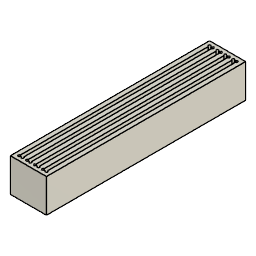
PCB Tolerance Tester (Autodesk Fusion 360 design; units mm, degrees)
Autodesk Fusion 360 part; units mm, degrees
sketch "Sketch1" plane through (0, 0, 0) normal (0, 0, 1) x (1, 0, 0)
  arc A0 (-0.5916, 85.05) -> (-0.493, 85.1333) centre (-0.5916, 85.15) ccw
  line L0 (-0.5916, 85.05) -> (-0.9084, 85.05)
  arc A1 (-1.007, 85.1333) -> (-1.5833, 84.557) centre (-1.5, 85.05) ccw
  arc A2 (0.0833, 84.557) -> (-0.493, 85.1333) centre (0, 85.05) ccw
  arc A3 (-1.007, 85.1333) -> (-0.9084, 85.05) centre (-0.9084, 85.15) ccw
  arc A4 (-1.5, 84.4584) -> (-1.5833, 84.557) centre (-1.6, 84.4584) ccw
  line L1 (-1.5, 84.4584) -> (-1.5, 0.5916)
  line L2 (0, 0.5916) -> (0, 84.4584)
  arc A5 (0.0833, 84.557) -> (0, 84.4584) centre (0.1, 84.4584) ccw
  line L3 (-1.5, 42.525) -> (0, 42.525) construction
  arc A6 (0, 0.5916) -> (0.0833, 0.493) centre (0.1, 0.5916) ccw
  arc A7 (-1.5833, 0.493) -> (-1.5, 0.5916) centre (-1.6, 0.5916) ccw
  arc A8 (-0.9084, 0) -> (-1.007, -0.0833) centre (-0.9084, -0.1) ccw
  arc A9 (-1.5833, 0.493) -> (-1.007, -0.0833) centre (-1.5, 0) ccw
  line L4 (-0.5916, 0) -> (-0.9084, 0)
  arc A10 (-0.493, -0.0833) -> (-0.5916, 0) centre (-0.5916, -0.1) ccw
  arc A11 (-0.493, -0.0833) -> (0.0833, 0.493) centre (0, 0) ccw
  line L5 (-3.5, 87.05) -> (12.65, 87.05)
  line L6 (12.65, 87.05) -> (12.65, -2)
  line L7 (12.65, -2) -> (-3.5, -2)
  line L8 (-3.5, -2) -> (-3.5, 87.05)
  line L9 (2.9334, 0) -> (2.5916, 0)
  line L10 (2, 84.4584) -> (2, 0.5916)
  arc A12 (3.6083, 84.557) -> (3.525, 84.4584) centre (3.625, 84.4584) ccw
  arc A13 (2.9334, 85.05) -> (3.032, 85.1333) centre (2.9334, 85.15) ccw
  arc A14 (1.9167, 0.493) -> (2.493, -0.0833) centre (2, 0) ccw
  arc A15 (2.493, 85.1333) -> (2.5916, 85.05) centre (2.5916, 85.15) ccw
  arc A16 (3.032, -0.0833) -> (3.6083, 0.493) centre (3.525, 0) ccw
  arc A17 (2, 84.4584) -> (1.9167, 84.557) centre (1.9, 84.4584) ccw
  arc A18 (3.525, 0.5916) -> (3.6083, 0.493) centre (3.625, 0.5916) ccw
  line L11 (2.9334, 85.05) -> (2.5916, 85.05)
  arc A19 (2.5916, 0) -> (2.493, -0.0833) centre (2.5916, -0.1) ccw
  line L12 (2, 42.525) -> (3.525, 42.525) construction
  arc A20 (2.493, 85.1333) -> (1.9167, 84.557) centre (2, 85.05) ccw
  arc A21 (3.6083, 84.557) -> (3.032, 85.1333) centre (3.525, 85.05) ccw
  arc A22 (3.032, -0.0833) -> (2.9334, 0) centre (2.9334, -0.1) ccw
  arc A23 (1.9167, 0.493) -> (2, 0.5916) centre (1.9, 0.5916) ccw
  line L13 (3.525, 0.5916) -> (3.525, 84.4584)
  arc A24 (5.4417, 0.493) -> (6.018, -0.0833) centre (5.525, 0) ccw
  line L14 (10.65, 0.5916) -> (10.65, 84.4584)
  line L15 (7.075, 0.5916) -> (7.075, 84.4584)
  line L16 (9.075, 42.525) -> (10.65, 42.525) construction
  arc A25 (9.568, 85.1333) -> (8.9917, 84.557) centre (9.075, 85.05) ccw
  line L17 (5.525, 84.4584) -> (5.525, 0.5916)
  arc A26 (6.582, -0.0833) -> (7.1583, 0.493) centre (7.075, 0) ccw
  arc A27 (10.157, -0.0833) -> (10.7333, 0.493) centre (10.65, 0) ccw
  arc A28 (6.018, 85.1333) -> (5.4417, 84.557) centre (5.525, 85.05) ccw
  line L18 (10.0584, 85.05) -> (9.6666, 85.05)
  arc A29 (8.9917, 0.493) -> (9.075, 0.5916) centre (8.975, 0.5916) ccw
  line L19 (6.4834, 0) -> (6.1166, 0)
  arc A30 (6.018, 85.1333) -> (6.1166, 85.05) centre (6.1166, 85.15) ccw
  arc A31 (9.568, 85.1333) -> (9.6666, 85.05) centre (9.6666, 85.15) ccw
  arc A32 (7.075, 0.5916) -> (7.1583, 0.493) centre (7.175, 0.5916) ccw
  line L20 (5.525, 42.525) -> (7.075, 42.525) construction
  arc A33 (6.1166, 0) -> (6.018, -0.0833) centre (6.1166, -0.1) ccw
  arc A34 (7.1583, 84.557) -> (7.075, 84.4584) centre (7.175, 84.4584) ccw
  line L21 (6.4834, 85.05) -> (6.1166, 85.05)
  arc A35 (9.075, 84.4584) -> (8.9917, 84.557) centre (8.975, 84.4584) ccw
  line L22 (9.075, 84.4584) -> (9.075, 0.5916)
  arc A36 (10.7333, 84.557) -> (10.65, 84.4584) centre (10.75, 84.4584) ccw
  arc A37 (6.582, -0.0833) -> (6.4834, 0) centre (6.4834, -0.1) ccw
  arc A38 (8.9917, 0.493) -> (9.568, -0.0833) centre (9.075, 0) ccw
  arc A39 (6.4834, 85.05) -> (6.582, 85.1333) centre (6.4834, 85.15) ccw
  arc A40 (7.1583, 84.557) -> (6.582, 85.1333) centre (7.075, 85.05) ccw
  arc A41 (9.6666, 0) -> (9.568, -0.0833) centre (9.6666, -0.1) ccw
  arc A42 (10.7333, 84.557) -> (10.157, 85.1333) centre (10.65, 85.05) ccw
  line L23 (10.0584, 0) -> (9.6666, 0)
  arc A43 (5.525, 84.4584) -> (5.4417, 84.557) centre (5.425, 84.4584) ccw
  arc A44 (10.65, 0.5916) -> (10.7333, 0.493) centre (10.75, 0.5916) ccw
  arc A45 (10.157, -0.0833) -> (10.0584, 0) centre (10.0584, -0.1) ccw
  arc A46 (5.4417, 0.493) -> (5.525, 0.5916) centre (5.425, 0.5916) ccw
  arc A47 (10.0584, 85.05) -> (10.157, 85.1333) centre (10.0584, 85.15) ccw
  arc A48 (9.568, 85.1333) -> (9.6666, 85.05) centre (9.6666, 85.15) ccw
  arc A49 (6.4834, 85.05) -> (6.582, 85.1333) centre (6.4834, 85.15) ccw
  arc A50 (10.0584, 85.05) -> (10.157, 85.1333) centre (10.0584, 85.15) ccw
  arc A51 (6.018, 85.1333) -> (5.4417, 84.557) centre (5.525, 85.05) ccw
  line L24 (10.0584, 85.05) -> (9.6666, 85.05)
  arc A52 (2.9334, 85.05) -> (3.032, 85.1333) centre (2.9334, 85.15) ccw
  arc A53 (10.7333, 84.557) -> (10.157, 85.1333) centre (10.65, 85.05) ccw
  arc A54 (6.018, 85.1333) -> (6.1166, 85.05) centre (6.1166, 85.15) ccw
  arc A55 (5.525, 84.4584) -> (5.4417, 84.557) centre (5.425, 84.4584) ccw
  arc A56 (2, 84.4584) -> (1.9167, 84.557) centre (1.9, 84.4584) ccw
  arc A57 (0.0833, 84.557) -> (0, 84.4584) centre (0.1, 84.4584) ccw
  arc A58 (10.7333, 84.557) -> (10.65, 84.4584) centre (10.75, 84.4584) ccw
  arc A59 (-1.007, 85.1333) -> (-1.5833, 84.557) centre (-1.5, 85.05) ccw
  line L25 (2.9334, 85.05) -> (2.5916, 85.05)
  arc A60 (3.6083, 84.557) -> (3.032, 85.1333) centre (3.525, 85.05) ccw
  arc A61 (-1.007, 85.1333) -> (-0.9084, 85.05) centre (-0.9084, 85.15) ccw
  arc A62 (7.1583, 84.557) -> (6.582, 85.1333) centre (7.075, 85.05) ccw
  arc A63 (2.493, 85.1333) -> (1.9167, 84.557) centre (2, 85.05) ccw
  arc A64 (9.075, 84.4584) -> (8.9917, 84.557) centre (8.975, 84.4584) ccw
  line L26 (-0.5916, 85.05) -> (-0.9084, 85.05)
  arc A65 (0.0833, 84.557) -> (-0.493, 85.1333) centre (0, 85.05) ccw
  arc A66 (-1.5, 84.4584) -> (-1.5833, 84.557) centre (-1.6, 84.4584) ccw
  arc A67 (-0.5916, 85.05) -> (-0.493, 85.1333) centre (-0.5916, 85.15) ccw
  arc A68 (7.1583, 84.557) -> (7.075, 84.4584) centre (7.175, 84.4584) ccw
  arc A69 (2.493, 85.1333) -> (2.5916, 85.05) centre (2.5916, 85.15) ccw
  line L27 (6.4834, 85.05) -> (6.1166, 85.05)
  arc A70 (3.6083, 84.557) -> (3.525, 84.4584) centre (3.625, 84.4584) ccw
  arc A71 (9.568, 85.1333) -> (8.9917, 84.557) centre (9.075, 85.05) ccw
  point P0 (-3.5, 87.05)
  point P1 (3.525, 0)
  point P2 (0.5, 87.05)
  point P3 (10.65, 0)
  point P4 (6.3, 0)
  dimension "d1" = 0.5
  dimension "d2" = 0.1
  dimension "d3" = 1.5
  dimension "d10" = 85.05
  dimension "d12" = 2
  dimension "d13" = 2
  dimension "d14" = 2
  dimension "d15" = 0.5
  dimension "d16" = 0.1
  dimension "d17" = 1.525
  dimension "d20" = 0.5
  dimension "d21" = 0.1
  dimension "d22" = 1.55
  dimension "d24" = 0.5
  dimension "d25" = 0.1
  dimension "d26" = 1.575
  dimension "d29" = 2
  dimension "d30" = 2
  dimension "d32" = 2
  dimension "d38" = 0.5
  dimension "d39" = 0.1
  dimension "d40" = 0.5
  dimension "d41" = 0.1
  dimension "d42" = 0.5
  dimension "d43" = 0.1
  dimension "d44" = 0.5
  dimension "d45" = 0.1
  dimension "d46" = 2
  constraint equal A1 A2
  constraint equal A3 A4
  constraint equal A0 A4
  constraint equal A4 A5
  constraint tangent L0 A3
  constraint tangent A1 A3
  constraint tangent A0 L0
  constraint tangent A0 A2
  constraint tangent A2 A5
  constraint tangent A1 A4
  constraint tangent A4 L1
  constraint tangent L2 A5
  constraint horizontal L0
  constraint vertical L1
  constraint horizontal A1.centre L0.end
  constraint horizontal A2.centre A0.start
  constraint vertical A2.centre L2.end
  constraint vertical A1.centre A4.start
  constraint vertical A11.centre L2.start
  constraint perpendicular L2 L3
  constraint midpoint L1 L3.start
  constraint midpoint L2 L3.end
  constraint symmetric L0.end L3 A8.start
  constraint symmetric A4.start L3 L1.end
  constraint symmetric A1.start L3 A8.end
  constraint symmetric A1.end L3 A7.start
  constraint symmetric A0.start L3 L4.start
  constraint symmetric L2.end L3 L2.start
  constraint symmetric A0.end L3 A10.start
  constraint symmetric A2.start L3 A6.end
  constraint symmetric A0 L3 A10
  constraint symmetric A1 L3 A9
  constraint symmetric A2 L3 A11
  constraint symmetric A3 L3 A8
  constraint symmetric A4 L3 A7
  constraint symmetric A5 L3 A6
  constraint horizontal A11.centre L4.start
  constraint horizontal L5
  constraint vertical L6
  constraint horizontal L7
  constraint vertical L8
  constraint equal A20 A21
  constraint equal A15 A17
  constraint equal A13 A17
  constraint equal A12 A17
  constraint tangent A15 L11
  constraint tangent A15 A20
  constraint tangent A13 L11
  constraint tangent A13 A21
  constraint tangent A12 A21
  constraint tangent A17 A20
  constraint tangent L10 A17
  constraint tangent A12 L13
  constraint horizontal L11
  constraint vertical L10
  constraint horizontal A15.end A20.centre
  constraint horizontal A13.start A21.centre
  constraint vertical A12.end A21.centre
  constraint vertical L10.start A20.centre
  constraint vertical A18.start P1
  constraint perpendicular L12 L13
  constraint midpoint L12.start L10
  constraint midpoint L12.end L13
  constraint symmetric A15.end L9.end L12
  constraint symmetric L10.start L10.end L12
  constraint symmetric A15.start A14.end L12
  constraint symmetric A17.end A14.start L12
  constraint symmetric A13.start L9.start L12
  constraint symmetric A12.end A18.start L12
  constraint symmetric A13.end A16.start L12
  constraint symmetric A16.end A12.start L12
  constraint symmetric A13 L12 A22
  constraint symmetric A14 L12 A20
  constraint symmetric A16 L12 A21
  constraint symmetric A15 A19 L12
  constraint symmetric A17 L12 A23
  constraint symmetric A12 A18 L12
  constraint horizontal P1 L9.start
  constraint equal A28 A40
  constraint equal A30 A43
  constraint equal A39 A43
  constraint equal A34 A43
  constraint tangent A30 L21
  constraint tangent A28 A30
  constraint tangent L21 A39
  constraint tangent A39 A40
  constraint tangent A34 A40
  constraint tangent A28 A43
  constraint tangent L17 A43
  constraint tangent L15 A34
  constraint horizontal L21
  constraint vertical L17
  constraint horizontal A30.end A28.centre
  constraint horizontal L21.start A40.centre
  constraint vertical L15.end A40.centre
  constraint vertical L17.start A28.centre
  constraint perpendicular L15 L20
  constraint midpoint L20.start L17
  constraint midpoint L20.end L15
  constraint symmetric A30.end L19.end L20
  constraint symmetric L17.start L17.end L20
  constraint symmetric A28.start A24.end L20
  constraint symmetric A28.end A24.start L20
  constraint symmetric L21.start L19.start L20
  constraint symmetric L15.end L15.start L20
  constraint symmetric A39.end A26.start L20
  constraint symmetric A26.end A34.start L20
  constraint symmetric L20 A37 A39
  constraint symmetric A24 A28 L20
  constraint symmetric A26 L20 A40
  constraint symmetric A30 L20 A33
  constraint symmetric L20 A43 A46
  constraint symmetric A32 L20 A34
  constraint equal A25 A42
  constraint equal A31 A35
  constraint equal A35 A47
  constraint equal A35 A36
  constraint tangent L18 A31
  constraint tangent A25 A31
  constraint tangent L18 A47
  constraint tangent A42 A47
  constraint tangent A36 A42
  constraint tangent A25 A35
  constraint tangent A35 L22
  constraint tangent L14 A36
  constraint horizontal L18
  constraint vertical L22
  constraint horizontal L18.end A25.centre
  constraint horizontal L18.start A42.centre
  constraint vertical L14.end A42.centre
  constraint vertical A35.start A25.centre
  constraint vertical L14.start P3
  constraint perpendicular L14 L16
  constraint midpoint L16.start L22
  constraint midpoint L16.end L14
  constraint symmetric L18.end A41.start L16
  constraint symmetric A35.start A29.end L16
  constraint symmetric A25.start A38.end L16
  constraint symmetric A25.end A29.start L16
  constraint symmetric L18.start L23.start L16
  constraint symmetric L14.end L14.start L16
  constraint symmetric A42.end A27.start L16
  constraint symmetric A27.end A36.start L16
  constraint symmetric L16 A45 A47
  constraint symmetric L16 A25 A38
  constraint symmetric L16 A27 A42
  constraint symmetric L16 A31 A41
  constraint symmetric L16 A29 A35
  constraint symmetric L16 A36 A44
  constraint horizontal P3 L23.start
  constraint midpoint P4 L19
  constraint collinear L4 L9
  constraint collinear L4 L19
  constraint collinear L4 L23
  constraint collinear L11 L21
  constraint collinear L0 L11
  constraint collinear L0 L18
  constraint equal A59 A65
  constraint equal A61 A66
  constraint equal A66 A67
  constraint equal A57 A66
  constraint tangent A61 L26
  constraint tangent A59 A61
  constraint tangent L26 A67
  constraint tangent A65 A67
  constraint tangent A57 A65
  constraint tangent A59 A66
  constraint horizontal L26
  constraint horizontal L0.end A1.centre
  constraint horizontal A0.start A2.centre
  constraint vertical L2.end A2.centre
  constraint vertical A4.start A1.centre
  constraint equal A60 A63
  constraint equal A56 A69
  constraint equal A52 A56
  constraint equal A56 A70
  constraint tangent L25 A69
  constraint tangent A63 A69
  constraint tangent A52 L25
  constraint tangent A52 A60
  constraint tangent A60 A70
  constraint tangent A56 A63
  constraint horizontal L25
  constraint equal A51 A62
  constraint equal A54 A55
  constraint equal A49 A55
  constraint equal A55 A68
  constraint tangent A54 L27
  constraint tangent A51 A54
  constraint tangent A49 L27
  constraint tangent A49 A62
  constraint tangent A62 A68
  constraint tangent A51 A55
  constraint horizontal L27
  constraint horizontal A28.centre A30.end
  constraint horizontal A40.centre L21.start
  constraint vertical A40.centre L15.end
  constraint vertical A28.centre L17.start
  constraint equal A53 A71
  constraint equal A48 A64
  constraint equal A50 A64
  constraint equal A58 A64
  constraint tangent A48 L24
  constraint tangent A48 A71
  constraint tangent A50 L24
  constraint tangent A50 A53
  constraint tangent A53 A58
  constraint tangent A64 A71
  constraint horizontal L24
  constraint horizontal A25.centre L18.end
  constraint horizontal A42.centre L18.start
  constraint vertical A42.centre L14.end
  constraint vertical A25.centre A35.start
  constraint collinear L25 L27
  constraint collinear L25 L26
  constraint collinear L24 L26
  measures "d1" radius of A1
  measures "d2" radius of A4
  measures "d3" distance of L1 L2
  measures "d10" distance of A11.centre L0
  measures "d12" distance of L4 L7
  measures "d13" distance of L1 L8
  measures "d14" distance of L0 L5
  measures "d15" radius of A20
  measures "d16" radius of A17
  measures "d17" distance of L10 L13
  measures "d20" radius of A28
  measures "d21" radius of A43
  measures "d22" distance of L15 L17
  measures "d24" radius of A25
  measures "d25" radius of A35
  measures "d26" distance of L14 L22
  measures "d29" distance of L13 L17
  measures "d30" distance of L15 L22
  measures "d32" distance of L2 L10
  measures "d38" radius of A59
  measures "d39" radius of A66
  measures "d40" radius of A63
  measures "d41" radius of A56
  measures "d42" radius of A51
  measures "d43" radius of A55
  measures "d44" radius of A71
  measures "d45" radius of A64
  measures "d46" distance of L6 L14
extrude "Extrude1" add sketch "Sketch1" along normal blind 14
sketch "Sketch2" plane through (0, 0, 0) normal (0, 0, -1) x (1, 0, 0)
  arc A0 (6.582, -85.1333) -> (7.1583, -84.557) centre (7.075, -85.05) ccw
  arc A1 (6.582, -85.1333) -> (6.4834, -85.05) centre (6.4834, -85.15) ccw
  line L0 (6.4834, -85.05) -> (6.1166, -85.05)
  arc A2 (6.1166, -85.05) -> (6.018, -85.1333) centre (6.1166, -85.15) ccw
  arc A3 (5.4417, -84.557) -> (6.018, -85.1333) centre (5.525, -85.05) ccw
  arc A4 (5.4417, -84.557) -> (5.525, -84.4584) centre (5.425, -84.4584) ccw
  line L1 (5.525, -84.4584) -> (5.525, -0.5916)
  arc A5 (5.525, -0.5916) -> (5.4417, -0.493) centre (5.425, -0.5916) ccw
  arc A6 (6.018, 0.0833) -> (5.4417, -0.493) centre (5.525, 0) ccw
  arc A7 (6.018, 0.0833) -> (6.1166, 0) centre (6.1166, 0.1) ccw
  line L2 (6.1166, 0) -> (6.4834, 0)
  arc A8 (6.4834, 0) -> (6.582, 0.0833) centre (6.4834, 0.1) ccw
  arc A9 (7.1583, -0.493) -> (6.582, 0.0833) centre (7.075, 0) ccw
  arc A10 (7.1583, -0.493) -> (7.075, -0.5916) centre (7.175, -0.5916) ccw
  line L3 (7.075, -0.5916) -> (7.075, -84.4584)
  arc A11 (7.075, -84.4584) -> (7.1583, -84.557) centre (7.175, -84.4584) ccw
  line L4 (10.0584, -85.05) -> (9.6666, -85.05)
  arc A12 (9.6666, -85.05) -> (9.568, -85.1333) centre (9.6666, -85.15) ccw
  arc A13 (8.9917, -84.557) -> (9.568, -85.1333) centre (9.075, -85.05) ccw
  arc A14 (8.9917, -84.557) -> (9.075, -84.4584) centre (8.975, -84.4584) ccw
  line L5 (9.075, -84.4584) -> (9.075, -0.5916)
  arc A15 (9.075, -0.5916) -> (8.9917, -0.493) centre (8.975, -0.5916) ccw
  arc A16 (9.568, 0.0833) -> (8.9917, -0.493) centre (9.075, 0) ccw
  arc A17 (9.568, 0.0833) -> (9.6666, 0) centre (9.6666, 0.1) ccw
  line L6 (9.6666, 0) -> (10.0584, 0)
  arc A18 (10.0584, 0) -> (10.157, 0.0833) centre (10.0584, 0.1) ccw
  arc A19 (10.7333, -0.493) -> (10.157, 0.0833) centre (10.65, 0) ccw
  arc A20 (10.7333, -0.493) -> (10.65, -0.5916) centre (10.75, -0.5916) ccw
  line L7 (10.65, -0.5916) -> (10.65, -84.4584)
  arc A21 (10.65, -84.4584) -> (10.7333, -84.557) centre (10.75, -84.4584) ccw
  arc A22 (10.157, -85.1333) -> (10.7333, -84.557) centre (10.65, -85.05) ccw
  arc A23 (10.157, -85.1333) -> (10.0584, -85.05) centre (10.0584, -85.15) ccw
  line L8 (2.9334, -85.05) -> (2.5916, -85.05)
  arc A24 (2.5916, -85.05) -> (2.493, -85.1333) centre (2.5916, -85.15) ccw
  arc A25 (1.9167, -84.557) -> (2.493, -85.1333) centre (2, -85.05) ccw
  arc A26 (1.9167, -84.557) -> (2, -84.4584) centre (1.9, -84.4584) ccw
  line L9 (2, -84.4584) -> (2, -0.5916)
  arc A27 (2, -0.5916) -> (1.9167, -0.493) centre (1.9, -0.5916) ccw
  arc A28 (2.493, 0.0833) -> (1.9167, -0.493) centre (2, 0) ccw
  arc A29 (2.493, 0.0833) -> (2.5916, 0) centre (2.5916, 0.1) ccw
  line L10 (2.5916, 0) -> (2.9334, 0)
  arc A30 (2.9334, 0) -> (3.032, 0.0833) centre (2.9334, 0.1) ccw
  arc A31 (3.6083, -0.493) -> (3.032, 0.0833) centre (3.525, 0) ccw
  arc A32 (3.6083, -0.493) -> (3.525, -0.5916) centre (3.625, -0.5916) ccw
  line L11 (3.525, -0.5916) -> (3.525, -84.4584)
  arc A33 (3.525, -84.4584) -> (3.6083, -84.557) centre (3.625, -84.4584) ccw
  arc A34 (3.032, -85.1333) -> (3.6083, -84.557) centre (3.525, -85.05) ccw
  arc A35 (3.032, -85.1333) -> (2.9334, -85.05) centre (2.9334, -85.15) ccw
  arc A36 (-1.5833, -84.557) -> (-1.007, -85.1333) centre (-1.5, -85.05) ccw
  arc A37 (-1.5833, -84.557) -> (-1.5, -84.4584) centre (-1.6, -84.4584) ccw
  line L12 (-1.5, -84.4584) -> (-1.5, -0.5916)
  arc A38 (-1.5, -0.5916) -> (-1.5833, -0.493) centre (-1.6, -0.5916) ccw
  arc A39 (-1.007, 0.0833) -> (-1.5833, -0.493) centre (-1.5, 0) ccw
  arc A40 (-1.007, 0.0833) -> (-0.9084, 0) centre (-0.9084, 0.1) ccw
  line L13 (-0.9084, 0) -> (-0.5916, 0)
  arc A41 (-0.5916, 0) -> (-0.493, 0.0833) centre (-0.5916, 0.1) ccw
  arc A42 (0.0833, -0.493) -> (-0.493, 0.0833) centre (0, 0) ccw
  arc A43 (0.0833, -0.493) -> (0, -0.5916) centre (0.1, -0.5916) ccw
  line L14 (0, -0.5916) -> (0, -84.4584)
  arc A44 (0, -84.4584) -> (0.0833, -84.557) centre (0.1, -84.4584) ccw
  arc A45 (-0.493, -85.1333) -> (0.0833, -84.557) centre (0, -85.05) ccw
  arc A46 (-0.493, -85.1333) -> (-0.5916, -85.05) centre (-0.5916, -85.15) ccw
  line L15 (-0.5916, -85.05) -> (-0.9084, -85.05)
  arc A47 (-0.9084, -85.05) -> (-1.007, -85.1333) centre (-0.9084, -85.15) ccw
  line L16 (12.65, 2) -> (-3.5, 2)
  line L17 (-3.5, 2) -> (-3.5, -87.05)
  line L18 (-3.5, -87.05) -> (12.65, -87.05)
  line L19 (12.65, -87.05) -> (12.65, 2)
  line L20 (12.65, -87.05) -> (-3.5, -87.05)
  line L21 (-3.5, -87.05) -> (-3.5, 2)
  line L22 (-3.5, 2) -> (12.65, 2)
  line L23 (12.65, 2) -> (12.65, -87.05)
  constraint horizontal L20
  constraint vertical L21
  constraint horizontal L22
  constraint vertical L23
  constraint coincident L16.end L17.start
  constraint coincident L18.end L19.start
extrude "Extrude2" add sketch "Sketch2" along normal blind 1 contours A0 A1 L0 A2 A3 A4 L1 A5 A6 A7 L2 A8 A9 A10 L3 A11 | L4 A12 A13 A14 L5 A15 A16 A17 L6 A18 A19 A20 L7 A21 A22 A23 | L8 A24 A25 A26 L9 A27 A28 A29 L10 A30 A31 A32 L11 A33 A34 A35 | A36 A37 L12 A38 A39 A40 L13 A41 A42 A43 L14 A44 A45 A46 L15 A47 | L16 L17 L18 L19 L20 L21 L22 L23
equation "d14 = d12"
equation "d26 = 1.55 mm + 0.025 mm"
equation "d29 = d13"
equation "d30 = d13"
equation "d32 = d13"
